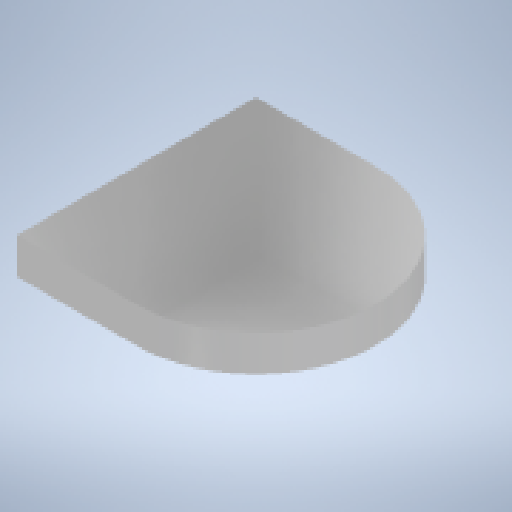
# Autodesk Inventor part: サイクロイドギア想定
Saved by Autodesk Inventor 2024 (Build 280153000, 153)
## iProperties
Created: 2023-05-31
Part Number: サイクロイドギア想定
Material: アルミニウム 6061
Document SubType Name: Modeling
Designer: yuta2
Mass: 2.89235 g
Surface Area: 9.28407 cm^2
Volume: 1.07124 cm^3
Density: 2.7 g/cm^3
Appearance: アルミニウム - フラット
Author: yuta2
Autodesk Inventor part; units mm, degrees
ref_plane "YZ Plane" through (0, 0, 0) normal (1, 0, 0) x (0, 1, 0)
ref_plane "XZ Plane" through (0, 0, 0) normal (0, 1, 0) x (-1, 0, 0)
ref_plane "XY Plane" through (0, 0, 0) normal (0, 0, 1) x (1, 0, 0)
sketch "スケッチ1" plane through (0, 0, 0) normal (0, 1, 0) x (-1, 0, 0)
  circle A0 centre (0, 0) radius 10
  dimension "d0" = 20
  constraints: 1 centre point, 1 coincident
  measures "d0" diameter of A0
extrude "押し出し1" add sketch "スケッチ1" along normal blind 3
sketch "スケッチ2" plane through (0, 3, 0) normal (0, 1, 0) x (1, 0, 0)
  circle A0 centre (0, 0) radius 10 projected
  line L0 (0, -10) -> (-10, -10)
  line L1 (-10, -10) -> (-10, 10)
  line L2 (-10, 10) -> (0, 10)
  line L3 (0, 10) -> (0, -10)
  circle A1 centre (0, 0) radius 10 projected
  point P0 (-10, 0)
  constraints: 8 end point, 2 horizontal, 2 parallel, 1 perpendicular, 1 tangent, 1 vertical, 2 other
extrude "押し出し2" add sketch "スケッチ2" against normal blind 3 contours A0 L1 L2 | L0 L1 A0
